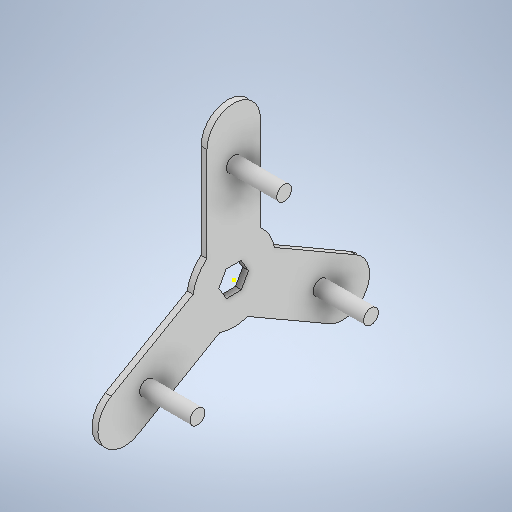
# Autodesk Inventor part: Porta_Satelite
Saved by Autodesk Inventor 2025.3 (Build 293356030, 356C)
## iProperties
Created: 2026-09-08
Part Number: Porta_Satelite
Material: Genérico
Document SubType Name: Modeling
Designer: marcu
Density: 1 g/cm^3
Appearance: Padrão
Author: marcu
Autodesk Inventor part; units mm, degrees
note: some values were not read from the file. Left out: dimensions or parameters whose unit could not be read.
ref_plane "YZ Plane" through (0, 0, 0) normal (1, 0, 0) x (0, 1, 0)
ref_plane "XZ Plane" through (0, 0, 0) normal (0, 1, 0) x (-1, 0, 0)
ref_plane "XY Plane" through (0, 0, 0) normal (0, 0, 1) x (1, 0, 0)
sketch "Esboço1" plane through (0, 0, 0) normal (1, 0, 0) x (0, 1, 0)
  circle A0 centre (0, 0) radius 51.5625
  dimension "d0" = 103.125
  constraints: 1 centre point, 1 coincident
  measures "d0" diameter of A0
extrude "Extrusão1" add sketch "Esboço1" along normal blind 2
sketch "Esboço2" plane through (2, 0, 0) normal (1, 0, 0) x (0, 0, -1)
  point P0 (0, 0)
sketch "Esboço3" plane through (2, 0, 0) normal (1, 0, 0) x (0, 0, -1)
  line L0 (-44.5522, -25.7222) -> (-12.0542, -6.9595)
  line L1 (12.0542, -6.9595) -> (44.5522, -25.7222)
  line L2 (0, 13.919) -> (0, 51.4445)
  circle A0 centre (0, 0) radius 51.4445
  circle A1 centre (0, 0) radius 33.75
  circle A2 centre (0, 0) radius 51.5625 projected
  line L3 (-44.5522, -25.7222) -> (0, 0) construction
  line L4 (-32.2394, -29.0214) -> (-4.6786, -13.1092)
  line L5 (-13.6921, 2.5028) -> (-41.253, -13.4095)
  arc A3 (-41.253, -13.4095) -> (-32.2394, -29.0214) centre (-36.7462, -21.2154) ccw
  line L6 (0, 13.919) -> (0, 51.4445)
  line L7 (0, 0) -> (0, 51.4445) construction
  line L8 (9.0136, 10.6063) -> (9.0136, 42.4309)
  line L9 (-9.0136, 42.4309) -> (-9.0136, 10.6063)
  arc A4 (9.0136, 42.4309) -> (-9.0136, 42.4309) centre (0, 42.4309) ccw
  line L10 (12.0542, -6.9595) -> (44.5522, -25.7222)
  line L11 (0, 0) -> (44.5522, -25.7222) construction
  line L12 (4.6786, -13.1092) -> (32.2394, -29.0214)
  line L13 (41.253, -13.4095) -> (13.6921, 2.5028)
  arc A5 (32.2394, -29.0214) -> (41.253, -13.4095) centre (36.7462, -21.2154) ccw
  arc A6 (-9.0136, 10.6063) -> (-13.6921, 2.5028) centre (0, 0) ccw
  arc A7 (-4.6786, -13.1092) -> (4.6786, -13.1092) centre (0, 0) ccw
  arc A8 (13.6921, 2.5028) -> (9.0136, 10.6063) centre (0, 0) ccw
  circle A9 centre (0, 33.75) radius 2.5
  circle A10 centre (29.2284, -16.875) radius 2.5
  circle A11 centre (-29.2284, -16.875) radius 2.5
  point P0 (-22.2761, -12.8611)
  point P1 (0, 51.4445)
  point P2 (0, 25.7222)
  point P3 (44.5522, -25.7222)
  point P4 (22.2761, -12.8611)
  dimension "d5" = 5
  dimension "d6" = 5
  dimension "d7" = 5
  dimension "d8" = 103.125
  dimension "d9" = 67.5
  constraints: 34 end point, 22 point on circle, 11 centre point, 6 coincident, 6 point on line, 6 tangent, 3 collinear, 3 midpoint, 3 parallel, 1 vertical
  measures "d5" diameter of A11
  measures "d6" diameter of A9
  measures "d7" diameter of A10
  measures "d8" diameter of A2
  measures "d9" diameter of A1
extrude "Extrusão2" cut sketch "Esboço3" against normal blind 2 contours A3 L5 A1 A11 L0 | L0 A11 A1 L4 A3 | A11 A1 L0 | L0 A1 A11 | A4 L8 A1 A9 L2 | L2 A9 A1 L9 A4 | A5 L12 A1 A10 L1 | L1 A10 A1 L13 A5 | A1 A11 L0 | L0 A11 A1 | A1 L5 A6 L9 A9 L8 A8 L13 A10 L12 A7 L4 A11 | A9 A1 L2 | L2 A1 A9 | A10 A1 L1 | L1 A1 A10 | A1 A9 L2 | L2 A9 A1 | A1 A10 L1 | L1 A10 A1 keep common part
sketch "Esboço4" plane through (2, 0, 0) normal (1, 0, 0) x (0, 0, -1)
  circle A0 centre (0, 0) radius 33.75
  circle A1 centre (0, 33.75) radius 2.5
  circle A2 centre (-29.2284, -16.875) radius 2.5
  circle A3 centre (29.2284, -16.875) radius 2.5
  dimension "d10" = 67.5
  dimension "d11" = 5
  dimension "d14" = 360
  constraints: 3 centre point, 1 coincident, 1 vertical alignment, 9 other
  measures "d11" diameter of A1
extrude "Extrusão3" add sketch "Esboço4" along normal blind 17 contours A1 A0 | A0 A1 | A3 A0 | A0 A3 | A2 A0 | A0 A2
sketch "Esboço5" plane through (0, 0, 0) normal (-1, 0, 0) x (0, 0, 1)
  line L0 (5, -0.0957) -> (2.4171, -4.378)
  line L1 (2.4171, -4.378) -> (-2.5829, -4.2823)
  line L2 (-2.5829, -4.2823) -> (-5, 0.0957)
  line L3 (-5, 0.0957) -> (-2.4171, 4.378)
  line L4 (-2.4171, 4.378) -> (2.5829, 4.2823)
  line L5 (2.5829, 4.2823) -> (5, -0.0957)
  point P0 (0, 0)
  dimension "d18" = 10
  constraints: 12 end point, 13 other
  measures "d18" horizontal distance of L0.start L2.end
extrude "Extrusão4" cut sketch "Esboço5" against normal blind 17
equation "\"d5\" = D_Furo_Planeta"
equation "\"d6\" = D_Furo_Planeta"
equation "\"d7\" = D_Furo_Planeta"
equation "\"d11\" = D_Furo_Planeta"
equation "\"modulo\" = 1.5"
equation "\"delta\" = 0.3"
equation "\"D_Furo_Sol\" = 8"
equation "\"D_Furo_Planeta\" = 5"
equation "\"Rendimento_eta\" = 0.85"
equation "\"Teste_Montagem\" = 0"
